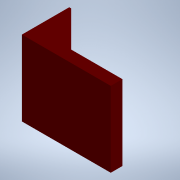
# Autodesk Inventor part: LPS_base
Saved by Autodesk Inventor 2022 (Build 260153000, 153)
## iProperties
Created: 2024-07-06
Part Number: LPS_base
Material: Типовые
Document SubType Name: Modeling
Designer: Капустяник Андрей
Density: 1 g/cm^3
Appearance: По умолчанию
Author: Капустяник Андрей
Autodesk Inventor part; units mm, degrees
ref_plane "YZ Plane" through (0, 0, 0) normal (1, 0, 0) x (0, 1, 0)
ref_plane "XZ Plane" through (0, 0, 0) normal (0, 1, 0) x (-1, 0, 0)
ref_plane "XY Plane" through (0, 0, 0) normal (0, 0, 1) x (1, 0, 0)
sketch "Эскиз1" plane through (0, 0, 0) normal (0, 0, 1) x (1, 0, 0)
  line L0 (28.51, -53.225) -> (-28.51, -53.225) projected
  line L1 (28.51, 53.225) -> (28.51, -53.225) projected
  line L2 (-28.51, 53.225) -> (28.51, 53.225) projected
  line L3 (-28.51, -53.225) -> (-28.51, 53.225) projected
  circle A0 centre (-23.7, 49.095) radius 2 projected
  circle A1 centre (-23.7, -49.095) radius 2 projected
  circle A2 centre (23.7, -49.095) radius 2 projected
  circle A3 centre (23.7, 49.095) radius 2 projected
  line L4 (-30.51, 55) -> (30.51, 55)
  line L5 (30.51, 55) -> (30.51, -55)
  line L6 (30.51, -55) -> (-30.51, -55)
  line L7 (-30.51, -55) -> (-30.51, 55)
  line L8 (-30.51, 55) -> (30.51, -55) construction
  line L9 (30.51, 55) -> (-30.51, -55) construction
  line L10 (-33.51, 58) -> (33.51, 58)
  line L11 (33.51, 58) -> (33.51, -58)
  line L12 (33.51, -58) -> (-33.51, -58)
  line L13 (-33.51, -58) -> (-33.51, 58)
  line L14 (30.51, 55) -> (100.51, 55)
  line L15 (100.51, 55) -> (100.51, -55)
  line L16 (100.51, -55) -> (30.51, -55)
  line L17 (33.51, -58) -> (103.51, -58)
  line L18 (103.51, -58) -> (103.51, 58)
  line L19 (103.51, 58) -> (33.51, 58)
  point P0 (0, 0)
  dimension "d0" = 110
  dimension "d1" = 2
  dimension "d2" = 3
  dimension "d3" = 70
  dimension "d4" = 70
  constraints: 32 end point, 6 parallel, 6 perpendicular, 2 midpoint, 1 horizontal, 3 other
  measures "d0" distance of L4.end L5.end
  measures "d1" distance between parallel lines of L3 L7
  measures "d2" distance between parallel lines of L7 L13
  measures "d3" distance of L4.end L14.end
  measures "d4" distance of L11.end L17.end
extrude "Выдавливание1" add sketch "Эскиз1" along normal blind 3 contours L0 L3 L2 L1 | A0 | A1 | A2 | A3 | L7 L6 L16 L11 L12 L13 L10 L14 L4 | L4 L5 L6 L7 | L14 L11 L16 L5 | L14 L15 L16 L11 | L11 L19 L18 L17 L16 L15 L14
sketch "Эскиз2" plane through (0, 0, 0) normal (0, 0, -1) x (-1, 0, 0)
  line L0 (-103.51, -58) -> (-103.51, 58) projected
  line L1 (33.51, -58) -> (-103.51, -58) projected
  line L2 (33.51, 58) -> (33.51, -58) projected
  line L3 (-103.51, 58) -> (33.51, 58) projected
  line L4 (-100.51, -55) -> (-100.51, 55)
  line L5 (-100.51, 55) -> (30.51, 55)
  line L6 (30.51, 55) -> (30.51, -55)
  line L7 (30.51, -55) -> (-100.51, -55)
  point P0 (0, 0)
  dimension "d7" = 3
  constraints: 8 end point, 3 other
  measures "d7" distance between parallel lines of L1 L7
extrude "Выдавливание2" add sketch "Эскиз2" along normal blind 70
sketch "Эскиз3" plane through (-33.51, 58, 3) normal (0, 1, 0) x (1, 0, 0)
  line L0 (3, 3) -> (3, 73) projected
  line L1 (3, 73) -> (73, 3)
  line L2 (3, 3) -> (134.02, 3) projected
  line L3 (0, 73) -> (0, 0) projected
  line L4 (137.02, 0) -> (0, 0) projected
  line L5 (137.02, 73) -> (137.02, 0) projected
  line L6 (0, 73) -> (137.02, 73) projected
  line L7 (134.02, 3) -> (134.02, 73) projected
  line L8 (134.02, 3) -> (137.02, 3)
  line L9 (137.02, 73) -> (137.02, 0) projected
  line L10 (137.02, 3) -> (137.02, 18)
  line L11 (137.02, 0) -> (137.02, 73) projected
  line L12 (137.02, 18) -> (58, 18)
  point P0 (33.51, 3)
  dimension "d10" = 45
  dimension "d13" = 15
  constraints: 8 end point, 4 point on line, 2 perpendicular
  measures "d10" angle of L1 L2
  measures "d13" distance of L8.end L10.end
extrude "Выдавливание3" cut sketch "Эскиз3" against normal up to surface (116 mm away) contours L6 L7 L12 L1 | L6 L5 L12 L7
